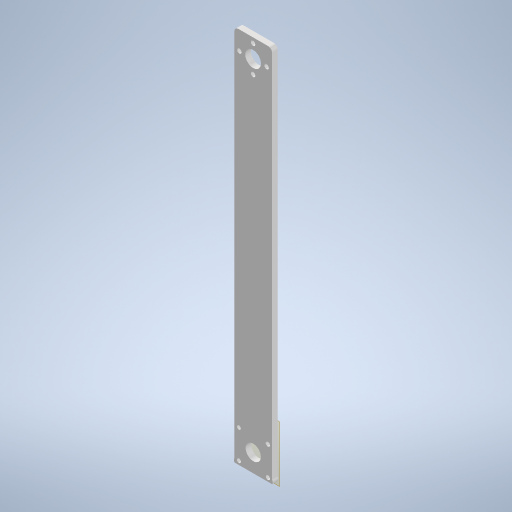
# Autodesk Inventor part: рука
Saved by Autodesk Inventor 2023 (Build 270158000, 158)
## iProperties
Created: 2025-02-02
Part Number: рука
Material: Типовые
Document SubType Name: Modeling
Designer: baranovaem
Density: 1 g/cm^3
Appearance: По умолчанию
Author: baranovaem
Autodesk Inventor part; units mm, degrees
ref_plane "YZ Plane" through (0, 0, 0) normal (1, 0, 0) x (0, 1, 0)
ref_plane "XZ Plane" through (0, 0, 0) normal (0, 1, 0) x (-1, 0, 0)
ref_plane "XY Plane" through (0, 0, 0) normal (0, 0, 1) x (1, 0, 0)
ref_plane "РабПлоскость1" through (0, 0, 0) normal (0, 0, 1) x (1, 0, 0)
sketch "Эскиз1" plane through (0, 0, 0) normal (0, 0, 1) x (1, 0, 0)
  line L0 (0.4175, 200.6086) -> (16.4175, 200.6086)
  line L1 (18.4175, 198.6086) -> (18.4175, 2.6086)
  line L2 (18.4175, 0.6086) -> (-1.5825, 0.6086)
  line L3 (-1.5825, 2.6086) -> (-1.5825, 198.6086)
  circle A0 centre (16.146, 17.8544) radius 1.1424
  circle A1 centre (16.1468, 2.552) radius 1.1415
  circle A2 centre (8.4175, 10.1937) radius 4.0638
  circle A3 centre (0.795, 2.6086) radius 1.0935
  circle A4 centre (0.7952, 17.8542) radius 1.0274
  line L4 (8.4175, 200.6086) -> (8.4175, 0.6086) construction
  arc A5 (18.4175, 0.6086) -> (18.4175, 2.6086) centre (16.6855, 1.6086) ccw
  arc A6 (-1.5825, 2.6086) -> (-1.5825, 0.6086) centre (0.1496, 1.6086) ccw
  circle A7 centre (8.3261, 183.6146) radius 1.1991 projected
  circle A8 centre (15.4815, 190.7279) radius 1.1951 projected
  circle A9 centre (8.3254, 197.9065) radius 1.1975 projected
  circle A10 centre (1.0262, 190.7251) radius 1.1979 projected
  circle A11 centre (8.3275, 190.7238) radius 4.2065 projected
  arc A12 (0.4175, 200.6086) -> (-1.5825, 198.6086) centre (0.4175, 198.6086) ccw
  arc A13 (18.4175, 198.6086) -> (16.4175, 200.6086) centre (16.4175, 198.6086) ccw
  point P0 (18.4175, 0.6086)
  point P1 (18.4175, 200.6086)
  point P2 (-1.5825, 0.6086)
  dimension "d0" = 200
  dimension "d1" = 20
  dimension "d3" = 2
  dimension "d4" = 2
  dimension "d5" = 2
  constraints: 10 end point, 9 centre point, 8 point on circle, 7 point on line, 4 tangent, 2 midpoint, 1 equal radius, 1 horizontal, 1 parallel, 1 perpendicular
  measures "d0" distance of point (18.418, 200.609) point (18.418, 0.609)
  measures "d1" distance of point (18.418, 0.609) point (-1.582, 0.609)
  measures "d3" distance from line of L2 A3.centre
  measures "d4" radius of A5
  measures "d5" radius of A12
extrude "Выдавливание1" add sketch "Эскиз1" along normal blind 3
